Autodesk Fusion 360 part; units mm, degrees
note: some values were not read from the file. Chosen so that the rebuilt part matches the saved one: which bodies a step acts on.
(part 2 of 3)
sketch "Sketch6" plane through (0, 0, 5) normal (0, 0, 1) x (-1, 0, 0)
  arc A0 (-101.6, 90) -> (-98.4, 90) centre (-100, 90) ccw
  line L0 (-101.6, 90) -> (-101.6, 94)
  arc A1 (-98.4, 94) -> (-101.6, 94) centre (-100, 94) ccw
  line L1 (-98.4, 94) -> (-98.4, 90)
  arc A2 (-110, 101.6) -> (-110, 98.4) centre (-110, 100) ccw
  line L2 (-110, 101.6) -> (-106, 101.6)
  arc A3 (-106, 98.4) -> (-106, 101.6) centre (-106, 100) ccw
  line L3 (-106, 98.4) -> (-110, 98.4)
  arc A4 (-90, 98.4) -> (-90, 101.6) centre (-90, 100) ccw
  line L4 (-90, 98.4) -> (-94, 98.4)
  arc A5 (-94, 101.6) -> (-94, 98.4) centre (-94, 100) ccw
  line L5 (-94, 101.6) -> (-90, 101.6)
  circle A6 centre (-100, 100) radius 3
  arc A7 (-98.4, 110) -> (-101.6, 110) centre (-100, 110) ccw
  line L6 (-98.4, 110) -> (-98.4, 106)
  arc A8 (-101.6, 106) -> (-98.4, 106) centre (-100, 106) ccw
  line L7 (-101.6, 106) -> (-101.6, 110)
  arc A9 (-30, -25) -> (-24, -25) centre (-27, -25) ccw
  line L8 (-30, -25) -> (-30, 25)
  arc A10 (-24, 25) -> (-30, 25) centre (-27, 25) ccw
  line L9 (-24, 25) -> (-24, -25)
  arc A11 (-17.7956, -15.5328) -> (-15.5328, -17.7956) centre (-16.6642, -16.6642) ccw
  line L10 (-17.7956, -15.5328) -> (-14.9672, -12.7044)
  arc A12 (-12.7044, -14.9672) -> (-14.9672, -12.7044) centre (-13.8358, -13.8358) ccw
  line L11 (-12.7044, -14.9672) -> (-15.5328, -17.7956)
  line L12 (12.7044, 14.9672) -> (15.5328, 17.7956)
  arc A13 (17.7956, 15.5328) -> (15.5328, 17.7956) centre (16.6642, 16.6642) ccw
  line L13 (17.7956, 15.5328) -> (14.9672, 12.7044)
  arc A14 (12.7044, 14.9672) -> (14.9672, 12.7044) centre (13.8358, 13.8358) ccw
  line L14 (14.9672, -12.7044) -> (17.7956, -15.5328)
  arc A15 (15.5328, -17.7956) -> (17.7956, -15.5328) centre (16.6642, -16.6642) ccw
  line L15 (15.5328, -17.7956) -> (12.7044, -14.9672)
  arc A16 (14.9672, -12.7044) -> (12.7044, -14.9672) centre (13.8358, -13.8358) ccw
  arc A17 (24, -25) -> (30, -25) centre (27, -25) ccw
  line L16 (24, -25) -> (24, 25)
  arc A18 (30, 25) -> (24, 25) centre (27, 25) ccw
  line L17 (30, 25) -> (30, -25)
  line L18 (-14.9672, 12.7044) -> (-17.7956, 15.5328)
  arc A19 (-15.5328, 17.7956) -> (-17.7956, 15.5328) centre (-16.6642, 16.6642) ccw
  line L19 (-15.5328, 17.7956) -> (-12.7044, 14.9672)
  arc A20 (-14.9672, 12.7044) -> (-12.7044, 14.9672) centre (-13.8358, 13.8358) ccw
  line L20 (112.7195, 117.7075) -> (119.1639, 120.4095)
  arc A21 (122.285, 116.8358) -> (119.1639, 120.4095) centre (120.1306, 118.104) ccw
  line L21 (122.285, 116.8358) -> (118.9823, 111.2253)
  arc A22 (116.8279, 109.9935) -> (118.9823, 111.2253) centre (116.8279, 112.4935) ccw
  line L22 (116.8279, 109.9935) -> (113.6861, 109.9935)
  arc A23 (111.1861, 112.4935) -> (113.6861, 109.9935) centre (113.6861, 112.4935) ccw
  line L23 (111.1861, 112.4935) -> (111.1861, 115.4019)
  arc A24 (112.7195, 117.7075) -> (111.1861, 115.4019) centre (113.6861, 115.4019) ccw
  arc A25 (101.6, 110) -> (98.4, 110) centre (100, 110) ccw
  line L24 (101.6, 110) -> (101.6, 106)
  arc A26 (98.4, 106) -> (101.6, 106) centre (100, 106) ccw
  line L25 (98.4, 106) -> (98.4, 110)
  circle A27 centre (100, 100) radius 3
  arc A28 (90, 101.6) -> (90, 98.4) centre (90, 100) ccw
  line L26 (90, 101.6) -> (94, 101.6)
  arc A29 (94, 98.4) -> (94, 101.6) centre (94, 100) ccw
  line L27 (94, 98.4) -> (90, 98.4)
  arc A30 (110, 98.4) -> (110, 101.6) centre (110, 100) ccw
  line L28 (110, 98.4) -> (106, 98.4)
  arc A31 (106, 101.6) -> (106, 98.4) centre (106, 100) ccw
  line L29 (106, 101.6) -> (110, 101.6)
  arc A32 (98.4, 90) -> (101.6, 90) centre (100, 90) ccw
  line L30 (98.4, 90) -> (98.4, 94)
  arc A33 (101.6, 94) -> (98.4, 94) centre (100, 94) ccw
  line L31 (101.6, 94) -> (101.6, 90)
  arc A34 (101.6, -90) -> (98.4, -90) centre (100, -90) ccw
  line L32 (101.6, -90) -> (101.6, -94)
  arc A35 (98.4, -94) -> (101.6, -94) centre (100, -94) ccw
  line L33 (98.4, -94) -> (98.4, -90)
  arc A36 (110, -101.6) -> (110, -98.4) centre (110, -100) ccw
  line L34 (110, -101.6) -> (106, -101.6)
  arc A37 (106, -98.4) -> (106, -101.6) centre (106, -100) ccw
  line L35 (106, -98.4) -> (110, -98.4)
  arc A38 (90, -98.4) -> (90, -101.6) centre (90, -100) ccw
  line L36 (90, -98.4) -> (94, -98.4)
  arc A39 (94, -101.6) -> (94, -98.4) centre (94, -100) ccw
  line L37 (94, -101.6) -> (90, -101.6)
  circle A40 centre (100, -100) radius 3
  arc A41 (98.4, -110) -> (101.6, -110) centre (100, -110) ccw
  line L38 (98.4, -110) -> (98.4, -106)
  arc A42 (101.6, -106) -> (98.4, -106) centre (100, -106) ccw
  line L39 (101.6, -106) -> (101.6, -110)
  line L40 (118.9823, -111.2253) -> (122.285, -116.8358)
  arc A43 (119.1639, -120.4095) -> (122.285, -116.8358) centre (120.1306, -118.104) ccw
  line L41 (119.1639, -120.4095) -> (112.7195, -117.7075)
  arc A44 (111.1861, -115.4019) -> (112.7195, -117.7075) centre (113.6861, -115.4019) ccw
  line L42 (111.1861, -115.4019) -> (111.1861, -112.4935)
  arc A45 (113.6861, -109.9935) -> (111.1861, -112.4935) centre (113.6861, -112.4935) ccw
  line L43 (113.6861, -109.9935) -> (116.8279, -109.9935)
  arc A46 (118.9823, -111.2253) -> (116.8279, -109.9935) centre (116.8279, -112.4935) ccw
  arc A47 (-101.6, -110) -> (-98.4, -110) centre (-100, -110) ccw
  line L44 (-101.6, -110) -> (-101.6, -106)
  arc A48 (-98.4, -106) -> (-101.6, -106) centre (-100, -106) ccw
  line L45 (-98.4, -106) -> (-98.4, -110)
  circle A49 centre (-100, -100) radius 3
  arc A50 (-90, -101.6) -> (-90, -98.4) centre (-90, -100) ccw
  line L46 (-90, -101.6) -> (-94, -101.6)
  arc A51 (-94, -98.4) -> (-94, -101.6) centre (-94, -100) ccw
  line L47 (-94, -98.4) -> (-90, -98.4)
  arc A52 (-110, -98.4) -> (-110, -101.6) centre (-110, -100) ccw
  line L48 (-110, -98.4) -> (-106, -98.4)
  arc A53 (-106, -101.6) -> (-106, -98.4) centre (-106, -100) ccw
  line L49 (-106, -101.6) -> (-110, -101.6)
  arc A54 (-98.4, -90) -> (-101.6, -90) centre (-100, -90) ccw
  line L50 (-98.4, -90) -> (-98.4, -94)
  arc A55 (-101.6, -94) -> (-98.4, -94) centre (-100, -94) ccw
  line L51 (-101.6, -94) -> (-101.6, -90)
  line L52 (-116.8279, -109.9935) -> (-113.6861, -109.9935)
  arc A56 (-111.1861, -112.4935) -> (-113.6861, -109.9935) centre (-113.6861, -112.4935) ccw
  line L53 (-111.1861, -112.4935) -> (-111.1861, -115.4019)
  arc A57 (-112.7195, -117.7075) -> (-111.1861, -115.4019) centre (-113.6861, -115.4019) ccw
  line L54 (-112.7195, -117.7075) -> (-119.1639, -120.4095)
  arc A58 (-122.285, -116.8358) -> (-119.1639, -120.4095) centre (-120.1306, -118.104) ccw
  line L55 (-122.285, -116.8358) -> (-118.9823, -111.2253)
  arc A59 (-116.8279, -109.9935) -> (-118.9823, -111.2253) centre (-116.8279, -112.4935) ccw
  line L56 (-118.9823, 111.2253) -> (-122.285, 116.8358)
  arc A60 (-119.1639, 120.4095) -> (-122.285, 116.8358) centre (-120.1306, 118.104) ccw
  line L57 (-119.1639, 120.4095) -> (-112.7195, 117.7075)
  arc A61 (-111.1861, 115.4019) -> (-112.7195, 117.7075) centre (-113.6861, 115.4019) ccw
  line L58 (-111.1861, 115.4019) -> (-111.1861, 112.4935)
  arc A62 (-113.6861, 109.9935) -> (-111.1861, 112.4935) centre (-113.6861, 112.4935) ccw
  line L59 (-113.6861, 109.9935) -> (-116.8279, 109.9935)
  arc A63 (-118.9823, 111.2253) -> (-116.8279, 109.9935) centre (-116.8279, 112.4935) ccw
  arc A64 (16.6527, -80.0321) -> (19.3611, -77.7595) centre (16.8706, -77.5416) ccw
  line L60 (19.3611, -77.7595) -> (21.3355, -55.1918)
  arc A65 (29.6477, -51.8989) -> (21.3355, -55.1918) centre (26.3165, -55.6276) ccw
  line L61 (29.6477, -51.8989) -> (81.7303, -98.4286)
  arc A66 (86.4985, -105.2878) -> (81.7303, -98.4286) centre (69.7381, -111.852) ccw
  arc A67 (86.4985, -105.2878) -> (94.5518, -113.4375) centre (100, -100) ccw
  line L62 (94.5518, -113.4375) -> (119.1307, -123.403)
  arc A68 (119.1307, -123.403) -> (125.4028, -116.3824) centre (121.0094, -118.7694) ccw
  line L63 (125.4028, -116.3824) -> (112.7409, -93.0776)
  arc A69 (112.7409, -93.0776) -> (103.7386, -85.9903) centre (100, -100) ccw
  arc A70 (96.3875, -82.0222) -> (103.7386, -85.9903) centre (108.3797, -68.5989) ccw
  line L64 (96.3875, -82.0222) -> (44.6753, -35.8235)
  arc A71 (38, -20.9087) -> (44.6753, -35.8235) centre (58, -20.9087) ccw
  line L65 (38, -20.9087) -> (38, 20.9087)
  arc A72 (44.6753, 35.8235) -> (38, 20.9087) centre (58, 20.9087) ccw
  line L66 (44.6753, 35.8235) -> (96.3875, 82.0222)
  arc A73 (103.7386, 85.9903) -> (96.3875, 82.0222) centre (108.3797, 68.5989) ccw
  arc A74 (103.7386, 85.9903) -> (112.7409, 93.0776) centre (100, 100) ccw
  line L67 (112.7409, 93.0776) -> (125.4028, 116.3824)
  arc A75 (125.4028, 116.3824) -> (119.1307, 123.403) centre (121.0094, 118.7694) ccw
  line L68 (119.1307, 123.403) -> (94.5518, 113.4375)
  arc A76 (94.5518, 113.4375) -> (86.4985, 105.2878) centre (100, 100) ccw
  arc A77 (81.7303, 98.4286) -> (86.4985, 105.2878) centre (69.7381, 111.852) ccw
  line L69 (81.7303, 98.4286) -> (29.156, 51.4596)
  arc A78 (20.8759, 54.4751) -> (29.156, 51.4596) centre (25.8248, 55.1883) ccw
  line L70 (20.8759, 54.4751) -> (16.1217, 87.466)
  arc A79 (16.1217, 87.466) -> (14.4465, 90.5321) centre (11.1729, 86.7528) ccw
  line L71 (14.4465, 90.5321) -> (10.4093, 94.0293)
  arc A80 (10.4093, 94.0293) -> (7.1356, 95.25) centre (7.1356, 90.25) ccw
  line L72 (7.1356, 95.25) -> (-7.1356, 95.25)
  arc A81 (-7.1356, 95.25) -> (-10.4093, 94.0293) centre (-7.1356, 90.25) ccw
  line L73 (-10.4093, 94.0293) -> (-14.4465, 90.5321)
  arc A82 (-14.4465, 90.5321) -> (-16.1217, 87.466) centre (-11.1729, 86.7528) ccw
  line L74 (-16.1217, 87.466) -> (-20.8759, 54.4751)
  arc A83 (-29.156, 51.4596) -> (-20.8759, 54.4751) centre (-25.8248, 55.1883) ccw
  line L75 (-29.156, 51.4596) -> (-81.7303, 98.4286)
  arc A84 (-86.4985, 105.2878) -> (-81.7303, 98.4286) centre (-69.7381, 111.852) ccw
  arc A85 (-86.4985, 105.2878) -> (-94.5518, 113.4375) centre (-100, 100) ccw
  line L76 (-94.5518, 113.4375) -> (-119.1307, 123.403)
  arc A86 (-119.1307, 123.403) -> (-125.4028, 116.3824) centre (-121.0094, 118.7694) ccw
  line L77 (-125.4028, 116.3824) -> (-112.7409, 93.0776)
  arc A87 (-112.7409, 93.0776) -> (-103.7386, 85.9903) centre (-100, 100) ccw
  arc A88 (-96.3875, 82.0222) -> (-103.7386, 85.9903) centre (-108.3797, 68.5989) ccw
  line L78 (-96.3875, 82.0222) -> (-44.6753, 35.8235)
  arc A89 (-38, 20.9087) -> (-44.6753, 35.8235) centre (-58, 20.9087) ccw
  line L79 (-38, 20.9087) -> (-38, -20.9087)
  arc A90 (-44.6753, -35.8235) -> (-38, -20.9087) centre (-58, -20.9087) ccw
  line L80 (-44.6753, -35.8235) -> (-96.3875, -82.0222)
  arc A91 (-103.7386, -85.9903) -> (-96.3875, -82.0222) centre (-108.3797, -68.5989) ccw
  arc A92 (-103.7386, -85.9903) -> (-112.7409, -93.0776) centre (-100, -100) ccw
  line L81 (-112.7409, -93.0776) -> (-125.4028, -116.3824)
  arc A93 (-125.4028, -116.3824) -> (-119.1307, -123.403) centre (-121.0094, -118.7694) ccw
  line L82 (-119.1307, -123.403) -> (-94.5518, -113.4375)
  arc A94 (-94.5518, -113.4375) -> (-86.4985, -105.2878) centre (-100, -100) ccw
  arc A95 (-81.7303, -98.4286) -> (-86.4985, -105.2878) centre (-69.7381, -111.852) ccw
  line L83 (-81.7303, -98.4286) -> (-29.6477, -51.8989)
  arc A96 (-21.3355, -55.1918) -> (-29.6477, -51.8989) centre (-26.3165, -55.6276) ccw
  line L84 (-21.3355, -55.1918) -> (-19.3611, -77.7595)
  arc A97 (-19.3611, -77.7595) -> (-16.6527, -80.0321) centre (-16.8706, -77.5416) ccw
  line L85 (-16.6527, -80.0321) -> (-12.2821, -79.6497)
  arc A98 (-12.2821, -79.6497) -> (-10.0175, -77.4546) centre (-12.5, -77.1592) ccw
  arc A99 (-7.535, -75.25) -> (-10.0175, -77.4546) centre (-7.535, -77.75) ccw
  line L86 (-7.535, -75.25) -> (7.535, -75.25)
  arc A100 (10.0175, -77.4546) -> (7.535, -75.25) centre (7.535, -77.75) ccw
  arc A101 (10.0175, -77.4546) -> (12.2821, -79.6497) centre (12.5, -77.1592) ccw
  line L87 (12.2821, -79.6497) -> (16.6527, -80.0321)
  line L88 (26, 35.4) -> (18, 35.4)
  arc A102 (18, 38.6) -> (18, 35.4) centre (18, 37) ccw
  line L89 (18, 38.6) -> (26, 38.6)
  arc A103 (26, 35.4) -> (26, 38.6) centre (26, 37) ccw
  circle A104 centre (14.8248, -75.7565) radius 1.6
  line L90 (-5, -61.3002) -> (5, -61.3002)
  arc A105 (5, -71.3002) -> (5, -61.3002) centre (5, -66.3002) ccw
  line L91 (5, -71.3002) -> (-5, -71.3002)
  arc A106 (-5, -61.3002) -> (-5, -71.3002) centre (-5, -66.3002) ccw
  circle A107 centre (16.4789, -56.85) radius 1.6
  line L92 (10, 39) -> (10, 36)
  arc A108 (4, 30) -> (10, 36) centre (4, 36) ccw
  line L93 (4, 30) -> (-4, 30)
  arc A109 (-10, 36) -> (-4, 30) centre (-4, 36) ccw
  line L94 (-10, 36) -> (-10, 39)
  arc A110 (-4, 45) -> (-10, 39) centre (-4, 39) ccw
  line L95 (-4, 45) -> (4, 45)
  arc A111 (10, 39) -> (4, 45) centre (4, 39) ccw
  line L96 (-26, 38.6) -> (-18, 38.6)
  arc A112 (-18, 35.4) -> (-18, 38.6) centre (-18, 37) ccw
  line L97 (-18, 35.4) -> (-26, 35.4)
  arc A113 (-26, 38.6) -> (-26, 35.4) centre (-26, 37) ccw
  circle A114 centre (-14.8248, -75.7565) radius 1.6
  line L98 (-12.5, -35.4) -> (12.5, -35.4)
  arc A115 (12.5, -38.6) -> (12.5, -35.4) centre (12.5, -37) ccw
  line L99 (12.5, -38.6) -> (-12.5, -38.6)
  arc A116 (-12.5, -35.4) -> (-12.5, -38.6) centre (-12.5, -37) ccw
  circle A117 centre (-16.4789, -56.85) radius 1.6
  line L100 (6, 80.25) -> (6, 60.25)
  arc A118 (-6, 60.25) -> (6, 60.25) centre (0, 60.25) ccw
  line L101 (-6, 60.25) -> (-6, 80.25)
  arc A119 (6, 80.25) -> (-6, 80.25) centre (0, 80.25) ccw
  line L102 (0, -61.3002) -> (0, -38.6) construction
  line L103 (5, -52.8369) -> (-5, -52.8369)
  line L104 (-5, -52.8369) -> (0, -44.1766)
  line L105 (5, -52.8369) -> (0, -44.1766)
  line L106 (2.5, -48.5067) -> (0, -49.9501)
  line L107 (-2.5, -48.5067) -> (0, -49.9501)
  line L108 (0, -52.8369) -> (0, -49.9501)
  dimension "d99" = 10
  constraint midpoint L90 L102.start
  constraint midpoint L99 L102.end
  constraint perpendicular L102 L103
  constraint coincident L102 L104.end
  constraint equal L103 L104
  constraint equal L103 L105
  constraint midpoint L105 L106.start
  constraint coincident L102 L106.end
  constraint perpendicular L105 L106
  constraint midpoint L104 L107.start
  constraint midpoint L103 L108.start
  constraint midpoint L102 L106.end
  measures "d99" distance of L103.start L103.end
extrude "Extrude6" cut sketch "Sketch6" against normal blind 5 contours L103 L105 L106 L108 | L103 L104 L107 L108 | L104 L105 L106 L107 bodies 2
chamfer "Chamfer2" distance 2 angle 45 3 edges at (-5, 52.8369, 2.5) (5, 52.8369, 2.5) (0, 44.1766, 2.5) on bodies 2
sketch "Sketch7" plane through (0, 0, 5) normal (0, 0, 1) x (-1, 0, 0)
  line L0 (6, 80.25) -> (6, 60.25)
  arc A0 (-6, 60.25) -> (6, 60.25) centre (0, 60.25) ccw
  line L1 (-6, 60.25) -> (-6, 80.25)
  arc A1 (6, 80.25) -> (-6, 80.25) centre (0, 80.25) ccw
  circle A2 centre (-16.4789, -56.85) radius 1.6
  line L2 (-12.5, -35.4) -> (12.5, -35.4)
  arc A3 (12.5, -38.6) -> (12.5, -35.4) centre (12.5, -37) ccw
  line L3 (12.5, -38.6) -> (-12.5, -38.6)
  arc A4 (-12.5, -35.4) -> (-12.5, -38.6) centre (-12.5, -37) ccw
  circle A5 centre (-14.8248, -75.7565) radius 1.6
  line L4 (-26, 38.6) -> (-18, 38.6)
  arc A6 (-18, 35.4) -> (-18, 38.6) centre (-18, 37) ccw
  line L5 (-18, 35.4) -> (-26, 35.4)
  arc A7 (-26, 38.6) -> (-26, 35.4) centre (-26, 37) ccw
  line L6 (10, 39) -> (10, 36)
  arc A8 (4, 30) -> (10, 36) centre (4, 36) ccw
  line L7 (4, 30) -> (-4, 30)
  arc A9 (-10, 36) -> (-4, 30) centre (-4, 36) ccw
  line L8 (-10, 36) -> (-10, 39)
  arc A10 (-4, 45) -> (-10, 39) centre (-4, 39) ccw
  line L9 (-4, 45) -> (4, 45)
  arc A11 (10, 39) -> (4, 45) centre (4, 39) ccw
  circle A12 centre (16.4789, -56.85) radius 1.6
  line L10 (-5, -61.3002) -> (5, -61.3002)
  arc A13 (5, -71.3002) -> (5, -61.3002) centre (5, -66.3002) ccw
  line L11 (5, -71.3002) -> (-5, -71.3002)
  arc A14 (-5, -61.3002) -> (-5, -71.3002) centre (-5, -66.3002) ccw
  circle A15 centre (14.8248, -75.7565) radius 1.6
  line L12 (26, 35.4) -> (18, 35.4)
  arc A16 (18, 38.6) -> (18, 35.4) centre (18, 37) ccw
  line L13 (18, 38.6) -> (26, 38.6)
  arc A17 (26, 35.4) -> (26, 38.6) centre (26, 37) ccw
  arc A18 (16.6527, -80.0321) -> (19.3611, -77.7595) centre (16.8706, -77.5416) ccw
  line L14 (19.3611, -77.7595) -> (21.3355, -55.1918)
  arc A19 (29.6477, -51.8989) -> (21.3355, -55.1918) centre (26.3165, -55.6276) ccw
  line L15 (29.6477, -51.8989) -> (81.7303, -98.4286)
  arc A20 (86.4985, -105.2878) -> (81.7303, -98.4286) centre (69.7381, -111.852) ccw
  arc A21 (86.4985, -105.2878) -> (94.5518, -113.4375) centre (100, -100) ccw
  line L16 (94.5518, -113.4375) -> (119.1307, -123.403)
  arc A22 (119.1307, -123.403) -> (125.4028, -116.3824) centre (121.0094, -118.7694) ccw
  line L17 (125.4028, -116.3824) -> (112.7409, -93.0776)
  arc A23 (112.7409, -93.0776) -> (103.7386, -85.9903) centre (100, -100) ccw
  arc A24 (96.3875, -82.0222) -> (103.7386, -85.9903) centre (108.3797, -68.5989) ccw
  line L18 (96.3875, -82.0222) -> (44.6753, -35.8235)
  arc A25 (38, -20.9087) -> (44.6753, -35.8235) centre (58, -20.9087) ccw
  line L19 (38, -20.9087) -> (38, 20.9087)
  arc A26 (44.6753, 35.8235) -> (38, 20.9087) centre (58, 20.9087) ccw
  line L20 (44.6753, 35.8235) -> (96.3875, 82.0222)
  arc A27 (103.7386, 85.9903) -> (96.3875, 82.0222) centre (108.3797, 68.5989) ccw
  arc A28 (103.7386, 85.9903) -> (112.7409, 93.0776) centre (100, 100) ccw
  line L21 (112.7409, 93.0776) -> (125.4028, 116.3824)
  arc A29 (125.4028, 116.3824) -> (119.1307, 123.403) centre (121.0094, 118.7694) ccw
  line L22 (119.1307, 123.403) -> (94.5518, 113.4375)
  arc A30 (94.5518, 113.4375) -> (86.4985, 105.2878) centre (100, 100) ccw
  arc A31 (81.7303, 98.4286) -> (86.4985, 105.2878) centre (69.7381, 111.852) ccw
  line L23 (81.7303, 98.4286) -> (29.156, 51.4596)
  arc A32 (20.8759, 54.4751) -> (29.156, 51.4596) centre (25.8248, 55.1883) ccw
  line L24 (20.8759, 54.4751) -> (16.1217, 87.466)
  arc A33 (16.1217, 87.466) -> (14.4465, 90.5321) centre (11.1729, 86.7528) ccw
  line L25 (14.4465, 90.5321) -> (10.4093, 94.0293)
  arc A34 (10.4093, 94.0293) -> (7.1356, 95.25) centre (7.1356, 90.25) ccw
  line L26 (7.1356, 95.25) -> (-7.1356, 95.25)
  arc A35 (-7.1356, 95.25) -> (-10.4093, 94.0293) centre (-7.1356, 90.25) ccw
  line L27 (-10.4093, 94.0293) -> (-14.4465, 90.5321)
  arc A36 (-14.4465, 90.5321) -> (-16.1217, 87.466) centre (-11.1729, 86.7528) ccw
  line L28 (-16.1217, 87.466) -> (-20.8759, 54.4751)
  arc A37 (-29.156, 51.4596) -> (-20.8759, 54.4751) centre (-25.8248, 55.1883) ccw
  line L29 (-29.156, 51.4596) -> (-81.7303, 98.4286)
  arc A38 (-86.4985, 105.2878) -> (-81.7303, 98.4286) centre (-69.7381, 111.852) ccw
  arc A39 (-86.4985, 105.2878) -> (-94.5518, 113.4375) centre (-100, 100) ccw
  line L30 (-94.5518, 113.4375) -> (-119.1307, 123.403)
  arc A40 (-119.1307, 123.403) -> (-125.4028, 116.3824) centre (-121.0094, 118.7694) ccw
  line L31 (-125.4028, 116.3824) -> (-112.7409, 93.0776)
  arc A41 (-112.7409, 93.0776) -> (-103.7386, 85.9903) centre (-100, 100) ccw
  arc A42 (-96.3875, 82.0222) -> (-103.7386, 85.9903) centre (-108.3797, 68.5989) ccw
  line L32 (-96.3875, 82.0222) -> (-44.6753, 35.8235)
  arc A43 (-38, 20.9087) -> (-44.6753, 35.8235) centre (-58, 20.9087) ccw
  line L33 (-38, 20.9087) -> (-38, -20.9087)
  arc A44 (-44.6753, -35.8235) -> (-38, -20.9087) centre (-58, -20.9087) ccw
  line L34 (-44.6753, -35.8235) -> (-96.3875, -82.0222)
  arc A45 (-103.7386, -85.9903) -> (-96.3875, -82.0222) centre (-108.3797, -68.5989) ccw
  arc A46 (-103.7386, -85.9903) -> (-112.7409, -93.0776) centre (-100, -100) ccw
  line L35 (-112.7409, -93.0776) -> (-125.4028, -116.3824)
  arc A47 (-125.4028, -116.3824) -> (-119.1307, -123.403) centre (-121.0094, -118.7694) ccw
  line L36 (-119.1307, -123.403) -> (-94.5518, -113.4375)
  arc A48 (-94.5518, -113.4375) -> (-86.4985, -105.2878) centre (-100, -100) ccw
  arc A49 (-81.7303, -98.4286) -> (-86.4985, -105.2878) centre (-69.7381, -111.852) ccw
  line L37 (-81.7303, -98.4286) -> (-29.6477, -51.8989)
  arc A50 (-21.3355, -55.1918) -> (-29.6477, -51.8989) centre (-26.3165, -55.6276) ccw
  line L38 (-21.3355, -55.1918) -> (-19.3611, -77.7595)
  arc A51 (-19.3611, -77.7595) -> (-16.6527, -80.0321) centre (-16.8706, -77.5416) ccw
  line L39 (-16.6527, -80.0321) -> (-12.2821, -79.6497)
  arc A52 (-12.2821, -79.6497) -> (-10.0175, -77.4546) centre (-12.5, -77.1592) ccw
  arc A53 (-7.535, -75.25) -> (-10.0175, -77.4546) centre (-7.535, -77.75) ccw
  line L40 (-7.535, -75.25) -> (7.535, -75.25)
  arc A54 (10.0175, -77.4546) -> (7.535, -75.25) centre (7.535, -77.75) ccw
  arc A55 (10.0175, -77.4546) -> (12.2821, -79.6497) centre (12.5, -77.1592) ccw
  line L41 (12.2821, -79.6497) -> (16.6527, -80.0321)
  line L42 (-118.9823, 111.2253) -> (-122.285, 116.8358)
  arc A56 (-119.1639, 120.4095) -> (-122.285, 116.8358) centre (-120.1306, 118.104) ccw
  line L43 (-119.1639, 120.4095) -> (-112.7195, 117.7075)
  arc A57 (-111.1861, 115.4019) -> (-112.7195, 117.7075) centre (-113.6861, 115.4019) ccw
  line L44 (-111.1861, 115.4019) -> (-111.1861, 112.4935)
  arc A58 (-113.6861, 109.9935) -> (-111.1861, 112.4935) centre (-113.6861, 112.4935) ccw
  line L45 (-113.6861, 109.9935) -> (-116.8279, 109.9935)
  arc A59 (-118.9823, 111.2253) -> (-116.8279, 109.9935) centre (-116.8279, 112.4935) ccw
  line L46 (-116.8279, -109.9935) -> (-113.6861, -109.9935)
  arc A60 (-111.1861, -112.4935) -> (-113.6861, -109.9935) centre (-113.6861, -112.4935) ccw
  line L47 (-111.1861, -112.4935) -> (-111.1861, -115.4019)
  arc A61 (-112.7195, -117.7075) -> (-111.1861, -115.4019) centre (-113.6861, -115.4019) ccw
  line L48 (-112.7195, -117.7075) -> (-119.1639, -120.4095)
  arc A62 (-122.285, -116.8358) -> (-119.1639, -120.4095) centre (-120.1306, -118.104) ccw
  line L49 (-122.285, -116.8358) -> (-118.9823, -111.2253)
  arc A63 (-116.8279, -109.9935) -> (-118.9823, -111.2253) centre (-116.8279, -112.4935) ccw
  arc A64 (-98.4, -90) -> (-101.6, -90) centre (-100, -90) ccw
  line L50 (-98.4, -90) -> (-98.4, -94)
  arc A65 (-101.6, -94) -> (-98.4, -94) centre (-100, -94) ccw
  line L51 (-101.6, -94) -> (-101.6, -90)
  arc A66 (-110, -98.4) -> (-110, -101.6) centre (-110, -100) ccw
  line L52 (-110, -98.4) -> (-106, -98.4)
  arc A67 (-106, -101.6) -> (-106, -98.4) centre (-106, -100) ccw
  line L53 (-106, -101.6) -> (-110, -101.6)
  arc A68 (-90, -101.6) -> (-90, -98.4) centre (-90, -100) ccw
  line L54 (-90, -101.6) -> (-94, -101.6)
  arc A69 (-94, -98.4) -> (-94, -101.6) centre (-94, -100) ccw
  line L55 (-94, -98.4) -> (-90, -98.4)
  circle A70 centre (-100, -100) radius 3
  arc A71 (-101.6, -110) -> (-98.4, -110) centre (-100, -110) ccw
  line L56 (-101.6, -110) -> (-101.6, -106)
  arc A72 (-98.4, -106) -> (-101.6, -106) centre (-100, -106) ccw
  line L57 (-98.4, -106) -> (-98.4, -110)
  line L58 (118.9823, -111.2253) -> (122.285, -116.8358)
  arc A73 (119.1639, -120.4095) -> (122.285, -116.8358) centre (120.1306, -118.104) ccw
  line L59 (119.1639, -120.4095) -> (112.7195, -117.7075)
  arc A74 (111.1861, -115.4019) -> (112.7195, -117.7075) centre (113.6861, -115.4019) ccw
  line L60 (111.1861, -115.4019) -> (111.1861, -112.4935)
  arc A75 (113.6861, -109.9935) -> (111.1861, -112.4935) centre (113.6861, -112.4935) ccw
  line L61 (113.6861, -109.9935) -> (116.8279, -109.9935)
  arc A76 (118.9823, -111.2253) -> (116.8279, -109.9935) centre (116.8279, -112.4935) ccw
  arc A77 (98.4, -110) -> (101.6, -110) centre (100, -110) ccw
  line L62 (98.4, -110) -> (98.4, -106)
  arc A78 (101.6, -106) -> (98.4, -106) centre (100, -106) ccw
  line L63 (101.6, -106) -> (101.6, -110)
  circle A79 centre (100, -100) radius 3
  arc A80 (90, -98.4) -> (90, -101.6) centre (90, -100) ccw
  line L64 (90, -98.4) -> (94, -98.4)
  arc A81 (94, -101.6) -> (94, -98.4) centre (94, -100) ccw
  line L65 (94, -101.6) -> (90, -101.6)
  arc A82 (110, -101.6) -> (110, -98.4) centre (110, -100) ccw
  line L66 (110, -101.6) -> (106, -101.6)
  arc A83 (106, -98.4) -> (106, -101.6) centre (106, -100) ccw
  line L67 (106, -98.4) -> (110, -98.4)
  arc A84 (101.6, -90) -> (98.4, -90) centre (100, -90) ccw
  line L68 (101.6, -90) -> (101.6, -94)
  arc A85 (98.4, -94) -> (101.6, -94) centre (100, -94) ccw
  line L69 (98.4, -94) -> (98.4, -90)
  arc A86 (98.4, 90) -> (101.6, 90) centre (100, 90) ccw
  line L70 (98.4, 90) -> (98.4, 94)
  arc A87 (101.6, 94) -> (98.4, 94) centre (100, 94) ccw
  line L71 (101.6, 94) -> (101.6, 90)
  arc A88 (110, 98.4) -> (110, 101.6) centre (110, 100) ccw
  line L72 (110, 98.4) -> (106, 98.4)
  arc A89 (106, 101.6) -> (106, 98.4) centre (106, 100) ccw
  line L73 (106, 101.6) -> (110, 101.6)
  arc A90 (90, 101.6) -> (90, 98.4) centre (90, 100) ccw
  line L74 (90, 101.6) -> (94, 101.6)
  arc A91 (94, 98.4) -> (94, 101.6) centre (94, 100) ccw
  line L75 (94, 98.4) -> (90, 98.4)
  circle A92 centre (100, 100) radius 3
  arc A93 (101.6, 110) -> (98.4, 110) centre (100, 110) ccw
  line L76 (101.6, 110) -> (101.6, 106)
  arc A94 (98.4, 106) -> (101.6, 106) centre (100, 106) ccw
  line L77 (98.4, 106) -> (98.4, 110)
  line L78 (112.7195, 117.7075) -> (119.1639, 120.4095)
  arc A95 (122.285, 116.8358) -> (119.1639, 120.4095) centre (120.1306, 118.104) ccw
  line L79 (122.285, 116.8358) -> (118.9823, 111.2253)
  arc A96 (116.8279, 109.9935) -> (118.9823, 111.2253) centre (116.8279, 112.4935) ccw
  line L80 (116.8279, 109.9935) -> (113.6861, 109.9935)
  arc A97 (111.1861, 112.4935) -> (113.6861, 109.9935) centre (113.6861, 112.4935) ccw
  line L81 (111.1861, 112.4935) -> (111.1861, 115.4019)
  arc A98 (112.7195, 117.7075) -> (111.1861, 115.4019) centre (113.6861, 115.4019) ccw
  line L82 (-14.9672, 12.7044) -> (-17.7956, 15.5328)
  arc A99 (-15.5328, 17.7956) -> (-17.7956, 15.5328) centre (-16.6642, 16.6642) ccw
  line L83 (-15.5328, 17.7956) -> (-12.7044, 14.9672)
  arc A100 (-14.9672, 12.7044) -> (-12.7044, 14.9672) centre (-13.8358, 13.8358) ccw
  arc A101 (24, -25) -> (30, -25) centre (27, -25) ccw
  line L84 (24, -25) -> (24, 25)
  arc A102 (30, 25) -> (24, 25) centre (27, 25) ccw
  line L85 (30, 25) -> (30, -25)
  line L86 (14.9672, -12.7044) -> (17.7956, -15.5328)
  arc A103 (15.5328, -17.7956) -> (17.7956, -15.5328) centre (16.6642, -16.6642) ccw
  line L87 (15.5328, -17.7956) -> (12.7044, -14.9672)
  arc A104 (14.9672, -12.7044) -> (12.7044, -14.9672) centre (13.8358, -13.8358) ccw
  line L88 (12.7044, 14.9672) -> (15.5328, 17.7956)
  arc A105 (17.7956, 15.5328) -> (15.5328, 17.7956) centre (16.6642, 16.6642) ccw
  line L89 (17.7956, 15.5328) -> (14.9672, 12.7044)
  arc A106 (12.7044, 14.9672) -> (14.9672, 12.7044) centre (13.8358, 13.8358) ccw
  arc A107 (-17.7956, -15.5328) -> (-15.5328, -17.7956) centre (-16.6642, -16.6642) ccw
  line L90 (-17.7956, -15.5328) -> (-14.9672, -12.7044)
  arc A108 (-12.7044, -14.9672) -> (-14.9672, -12.7044) centre (-13.8358, -13.8358) ccw
  line L91 (-12.7044, -14.9672) -> (-15.5328, -17.7956)
  arc A109 (-30, -25) -> (-24, -25) centre (-27, -25) ccw
  line L92 (-30, -25) -> (-30, 25)
  arc A110 (-24, 25) -> (-30, 25) centre (-27, 25) ccw
  line L93 (-24, 25) -> (-24, -25)
  arc A111 (-98.4, 110) -> (-101.6, 110) centre (-100, 110) ccw
  line L94 (-98.4, 110) -> (-98.4, 106)
  arc A112 (-101.6, 106) -> (-98.4, 106) centre (-100, 106) ccw
  line L95 (-101.6, 106) -> (-101.6, 110)
  circle A113 centre (-100, 100) radius 3
  arc A114 (-90, 98.4) -> (-90, 101.6) centre (-90, 100) ccw
  line L96 (-90, 98.4) -> (-94, 98.4)
  arc A115 (-94, 101.6) -> (-94, 98.4) centre (-94, 100) ccw
  line L97 (-94, 101.6) -> (-90, 101.6)
  arc A116 (-110, 101.6) -> (-110, 98.4) centre (-110, 100) ccw
  line L98 (-110, 101.6) -> (-106, 101.6)
  arc A117 (-106, 98.4) -> (-106, 101.6) centre (-106, 100) ccw
  line L99 (-106, 98.4) -> (-110, 98.4)
  arc A118 (-101.6, 90) -> (-98.4, 90) centre (-100, 90) ccw
  line L100 (-101.6, 90) -> (-101.6, 94)
  arc A119 (-98.4, 94) -> (-101.6, 94) centre (-100, 94) ccw
  line L101 (-98.4, 94) -> (-98.4, 90)
  line L102 (1, -45.9087) -> (4, -51.1048)
  line L103 (4, -51.1048) -> (3, -52.8369)
  line L104 (3, -52.8369) -> (-3, -52.8369)
  line L105 (-3, -52.8369) -> (-4, -51.1048)
  line L106 (-4, -51.1048) -> (-1, -45.9087)
  line L107 (-1, -45.9087) -> (1, -45.9087)
  line L108 (-8.6603, -5) -> (0, -10)
  line L109 (0, -10) -> (8.6603, -5)
  line L110 (8.6603, -5) -> (8.6603, 5)
  line L111 (8.6603, 5) -> (0, 10)
  line L112 (0, 10) -> (-8.6603, 5)
  line L113 (-8.6603, 5) -> (-8.6603, -5)
  line L114 (0, -10) -> (0, 0) construction
  line L115 (1.6, -11) -> (1.6, -9)
  arc A120 (1.6, -9) -> (-1.6, -9) centre (0, -9) ccw
  line L116 (-1.6, -9) -> (-1.6, -11)
  arc A121 (-1.6, -11) -> (1.6, -11) centre (0, -11) ccw
  line L117 (0, -11) -> (0, -9) construction
  arc A122 (8.7263, -6.8856) -> (10.3263, -4.1144) centre (9.5263, -5.5) ccw
  line L118 (10.3263, -4.1144) -> (8.5942, -3.1144)
  line L119 (6.9942, -5.8856) -> (8.7263, -6.8856)
  arc A123 (8.5942, -3.1144) -> (6.9942, -5.8856) centre (7.7942, -4.5) ccw
  arc A124 (10.3263, 4.1144) -> (8.7263, 6.8856) centre (9.5263, 5.5) ccw
  line L120 (8.7263, 6.8856) -> (6.9942, 5.8856)
  line L121 (8.5942, 3.1144) -> (10.3263, 4.1144)
  arc A125 (6.9942, 5.8856) -> (8.5942, 3.1144) centre (7.7942, 4.5) ccw
  arc A126 (1.6, 11) -> (-1.6, 11) centre (0, 11) ccw
  line L122 (-1.6, 11) -> (-1.6, 9)
  line L123 (1.6, 9) -> (1.6, 11)
  arc A127 (-1.6, 9) -> (1.6, 9) centre (0, 9) ccw
  arc A128 (-8.7263, 6.8856) -> (-10.3263, 4.1144) centre (-9.5263, 5.5) ccw
  line L124 (-10.3263, 4.1144) -> (-8.5942, 3.1144)
  line L125 (-6.9942, 5.8856) -> (-8.7263, 6.8856)
  arc A129 (-8.5942, 3.1144) -> (-6.9942, 5.8856) centre (-7.7942, 4.5) ccw
  arc A130 (-10.3263, -4.1144) -> (-8.7263, -6.8856) centre (-9.5263, -5.5) ccw
  line L126 (-8.7263, -6.8856) -> (-6.9942, -5.8856)
  line L127 (-8.5942, -3.1144) -> (-10.3263, -4.1144)
  arc A131 (-6.9942, -5.8856) -> (-8.5942, -3.1144) centre (-7.7942, -4.5) ccw
  point P0 (0, -10)
  dimension "d103" = 10
  dimension "d104" = 1
  dimension "d105" = 3.2
  dimension "d107" = 360
  constraint coincident L114.end origin
  constraint vertical L114
  constraint tangent L115 A120
  constraint tangent A120 L116
  constraint parallel L115 L116
  constraint tangent L116 A121
  constraint tangent L115 A121
  constraint coincident L114 A120.centre
  constraint parallel L114 L117
  constraint coincident P0 L108.end
  constraint midpoint L117 P0
  measures "d103" distance of L108.start L114.end
  measures "d104" distance of A120.centre P0
  measures "d105" diameter of A120
extrude "Extrude7" cut sketch "Sketch7" against normal blind 5 contours L108 L113 L126 L127 A131 | L108 L113 A130 L126 L127 | L108 L109 L110 L111 L112 L113 L115 A120 L116 L118 L119 A123 L120 L121 A125 L122 L123 A127 L124 L125 A129 L126 L127 A131 | L108 L109 L115 A120 L116 | L108 L109 L115 L116 A121 | L112 L113 A128 L124 L125 | L112 L113 L124 L125 A129 | L109 L110 L118 L119 A123 | L109 L110 A122 L118 L119 | L111 L112 A126 L122 L123 | L111 L112 L122 L123 A127 | L110 L111 L120 L121 A125 | L110 L111 A124 L120 L121 bodies 2
fillet "Fillet10" radius 2.5 12 edges at (-7.0603, 5.9238, 2.5) (-1.6, 9.0762, 2.5) (1.6, 9.0762, 2.5) (7.0603, 5.9238, 2.5) (8.6603, 3.1525, 2.5) (8.6603, -3.1525, 2.5) (7.0603, -5.9238, 2.5) (1.6, -9.0762, 2.5) (-1.6, -9.0762, 2.5) (-7.0603, -5.9238, 2.5) (-8.6603, -3.1525, 2.5) (-8.6603, 3.1525, 2.5) on bodies 2
sketch "Sketch8" plane through (0, 0, 5) normal (0, 0, 1) x (-1, 0, 0)
  arc A0 (8.6603, -1.7091) -> (9.9103, -3.8742) centre (11.1603, -1.7091) ccw
  line L0 (9.9103, -3.8742) -> (10.3263, -4.1144)
  arc A1 (8.7263, -6.8856) -> (10.3263, -4.1144) centre (9.5263, -5.5) ccw
  line L1 (8.7263, -6.8856) -> (8.3103, -6.6454)
  arc A2 (8.3103, -6.6454) -> (5.8103, -6.6454) centre (7.0603, -8.8105) ccw
  line L2 (5.8103, -6.6454) -> (2.85, -8.3546)
  arc A3 (2.85, -8.3546) -> (1.6, -10.5196) centre (4.1, -10.5196) ccw
  line L3 (1.6, -10.5196) -> (1.6, -11)
  arc A4 (-1.6, -11) -> (1.6, -11) centre (0, -11) ccw
  line L4 (-1.6, -11) -> (-1.6, -10.5196)
  arc A5 (-1.6, -10.5196) -> (-2.85, -8.3546) centre (-4.1, -10.5196) ccw
  line L5 (-2.85, -8.3546) -> (-5.8103, -6.6454)
  arc A6 (-5.8103, -6.6454) -> (-8.3103, -6.6454) centre (-7.0603, -8.8105) ccw
  line L6 (-8.3103, -6.6454) -> (-8.7263, -6.8856)
  arc A7 (-10.3263, -4.1144) -> (-8.7263, -6.8856) centre (-9.5263, -5.5) ccw
  line L7 (-10.3263, -4.1144) -> (-9.9103, -3.8742)
  arc A8 (-9.9103, -3.8742) -> (-8.6603, -1.7091) centre (-11.1603, -1.7091) ccw
  line L8 (-8.6603, -1.7091) -> (-8.6603, 1.7091)
  arc A9 (-8.6603, 1.7091) -> (-9.9103, 3.8742) centre (-11.1603, 1.7091) ccw
  line L9 (-9.9103, 3.8742) -> (-10.3263, 4.1144)
  arc A10 (-8.7263, 6.8856) -> (-10.3263, 4.1144) centre (-9.5263, 5.5) ccw
  line L10 (-8.7263, 6.8856) -> (-8.3103, 6.6454)
  arc A11 (-8.3103, 6.6454) -> (-5.8103, 6.6454) centre (-7.0603, 8.8105) ccw
  line L11 (-5.8103, 6.6454) -> (-2.85, 8.3546)
  arc A12 (-2.85, 8.3546) -> (-1.6, 10.5196) centre (-4.1, 10.5196) ccw
  line L12 (-1.6, 10.5196) -> (-1.6, 11)
  arc A13 (1.6, 11) -> (-1.6, 11) centre (0, 11) ccw
  line L13 (1.6, 11) -> (1.6, 10.5196)
  arc A14 (1.6, 10.5196) -> (2.85, 8.3546) centre (4.1, 10.5196) ccw
  line L14 (2.85, 8.3546) -> (5.8103, 6.6454)
  arc A15 (5.8103, 6.6454) -> (8.3103, 6.6454) centre (7.0603, 8.8105) ccw
  line L15 (8.3103, 6.6454) -> (8.7263, 6.8856)
  arc A16 (10.3263, 4.1144) -> (8.7263, 6.8856) centre (9.5263, 5.5) ccw
  line L16 (10.3263, 4.1144) -> (9.9103, 3.8742)
  arc A17 (9.9103, 3.8742) -> (8.6603, 1.7091) centre (11.1603, 1.7091) ccw
  line L17 (8.6603, 1.7091) -> (8.6603, -1.7091)
  line L18 (1, -45.9087) -> (4, -51.1048)
  line L19 (4, -51.1048) -> (3, -52.8369)
  line L20 (3, -52.8369) -> (-3, -52.8369)
  line L21 (-3, -52.8369) -> (-4, -51.1048)
  line L22 (-4, -51.1048) -> (-1, -45.9087)
  line L23 (-1, -45.9087) -> (1, -45.9087)
  arc A18 (-101.6, 90) -> (-98.4, 90) centre (-100, 90) ccw
  line L24 (-101.6, 90) -> (-101.6, 94)
  arc A19 (-98.4, 94) -> (-101.6, 94) centre (-100, 94) ccw
  line L25 (-98.4, 94) -> (-98.4, 90)
  arc A20 (-110, 101.6) -> (-110, 98.4) centre (-110, 100) ccw
  line L26 (-110, 101.6) -> (-106, 101.6)
  arc A21 (-106, 98.4) -> (-106, 101.6) centre (-106, 100) ccw
  line L27 (-106, 98.4) -> (-110, 98.4)
  arc A22 (-90, 98.4) -> (-90, 101.6) centre (-90, 100) ccw
  line L28 (-90, 98.4) -> (-94, 98.4)
  arc A23 (-94, 101.6) -> (-94, 98.4) centre (-94, 100) ccw
  line L29 (-94, 101.6) -> (-90, 101.6)
  circle A24 centre (-100, 100) radius 3
  arc A25 (-98.4, 110) -> (-101.6, 110) centre (-100, 110) ccw
  line L30 (-98.4, 110) -> (-98.4, 106)
  arc A26 (-101.6, 106) -> (-98.4, 106) centre (-100, 106) ccw
  line L31 (-101.6, 106) -> (-101.6, 110)
  arc A27 (-30, -25) -> (-24, -25) centre (-27, -25) ccw
  line L32 (-30, -25) -> (-30, 25)
  arc A28 (-24, 25) -> (-30, 25) centre (-27, 25) ccw
  line L33 (-24, 25) -> (-24, -25)
  arc A29 (-17.7956, -15.5328) -> (-15.5328, -17.7956) centre (-16.6642, -16.6642) ccw
  line L34 (-17.7956, -15.5328) -> (-14.9672, -12.7044)
  arc A30 (-12.7044, -14.9672) -> (-14.9672, -12.7044) centre (-13.8358, -13.8358) ccw
  line L35 (-12.7044, -14.9672) -> (-15.5328, -17.7956)
  line L36 (12.7044, 14.9672) -> (15.5328, 17.7956)
  arc A31 (17.7956, 15.5328) -> (15.5328, 17.7956) centre (16.6642, 16.6642) ccw
  line L37 (17.7956, 15.5328) -> (14.9672, 12.7044)
  arc A32 (12.7044, 14.9672) -> (14.9672, 12.7044) centre (13.8358, 13.8358) ccw
  line L38 (14.9672, -12.7044) -> (17.7956, -15.5328)
  arc A33 (15.5328, -17.7956) -> (17.7956, -15.5328) centre (16.6642, -16.6642) ccw
  line L39 (15.5328, -17.7956) -> (12.7044, -14.9672)
  arc A34 (14.9672, -12.7044) -> (12.7044, -14.9672) centre (13.8358, -13.8358) ccw
  arc A35 (24, -25) -> (30, -25) centre (27, -25) ccw
  line L40 (24, -25) -> (24, 25)
  arc A36 (30, 25) -> (24, 25) centre (27, 25) ccw
  line L41 (30, 25) -> (30, -25)
  line L42 (-14.9672, 12.7044) -> (-17.7956, 15.5328)
  arc A37 (-15.5328, 17.7956) -> (-17.7956, 15.5328) centre (-16.6642, 16.6642) ccw
  line L43 (-15.5328, 17.7956) -> (-12.7044, 14.9672)
  arc A38 (-14.9672, 12.7044) -> (-12.7044, 14.9672) centre (-13.8358, 13.8358) ccw
  line L44 (112.7195, 117.7075) -> (119.1639, 120.4095)
  arc A39 (122.285, 116.8358) -> (119.1639, 120.4095) centre (120.1306, 118.104) ccw
  line L45 (122.285, 116.8358) -> (118.9823, 111.2253)
  arc A40 (116.8279, 109.9935) -> (118.9823, 111.2253) centre (116.8279, 112.4935) ccw
  line L46 (116.8279, 109.9935) -> (113.6861, 109.9935)
  arc A41 (111.1861, 112.4935) -> (113.6861, 109.9935) centre (113.6861, 112.4935) ccw
  line L47 (111.1861, 112.4935) -> (111.1861, 115.4019)
  arc A42 (112.7195, 117.7075) -> (111.1861, 115.4019) centre (113.6861, 115.4019) ccw
  arc A43 (101.6, 110) -> (98.4, 110) centre (100, 110) ccw
  line L48 (101.6, 110) -> (101.6, 106)
  arc A44 (98.4, 106) -> (101.6, 106) centre (100, 106) ccw
  line L49 (98.4, 106) -> (98.4, 110)
  circle A45 centre (100, 100) radius 3
  arc A46 (90, 101.6) -> (90, 98.4) centre (90, 100) ccw
  line L50 (90, 101.6) -> (94, 101.6)
  arc A47 (94, 98.4) -> (94, 101.6) centre (94, 100) ccw
  line L51 (94, 98.4) -> (90, 98.4)
  arc A48 (110, 98.4) -> (110, 101.6) centre (110, 100) ccw
  line L52 (110, 98.4) -> (106, 98.4)
  arc A49 (106, 101.6) -> (106, 98.4) centre (106, 100) ccw
  line L53 (106, 101.6) -> (110, 101.6)
  arc A50 (98.4, 90) -> (101.6, 90) centre (100, 90) ccw
  line L54 (98.4, 90) -> (98.4, 94)
  arc A51 (101.6, 94) -> (98.4, 94) centre (100, 94) ccw
  line L55 (101.6, 94) -> (101.6, 90)
  arc A52 (101.6, -90) -> (98.4, -90) centre (100, -90) ccw
  line L56 (101.6, -90) -> (101.6, -94)
  arc A53 (98.4, -94) -> (101.6, -94) centre (100, -94) ccw
  line L57 (98.4, -94) -> (98.4, -90)
  arc A54 (110, -101.6) -> (110, -98.4) centre (110, -100) ccw
  line L58 (110, -101.6) -> (106, -101.6)
  arc A55 (106, -98.4) -> (106, -101.6) centre (106, -100) ccw
  line L59 (106, -98.4) -> (110, -98.4)
  arc A56 (90, -98.4) -> (90, -101.6) centre (90, -100) ccw
  line L60 (90, -98.4) -> (94, -98.4)
  arc A57 (94, -101.6) -> (94, -98.4) centre (94, -100) ccw
  line L61 (94, -101.6) -> (90, -101.6)
  circle A58 centre (100, -100) radius 3
  arc A59 (98.4, -110) -> (101.6, -110) centre (100, -110) ccw
  line L62 (98.4, -110) -> (98.4, -106)
  arc A60 (101.6, -106) -> (98.4, -106) centre (100, -106) ccw
  line L63 (101.6, -106) -> (101.6, -110)
  line L64 (118.9823, -111.2253) -> (122.285, -116.8358)
  arc A61 (119.1639, -120.4095) -> (122.285, -116.8358) centre (120.1306, -118.104) ccw
  line L65 (119.1639, -120.4095) -> (112.7195, -117.7075)
  arc A62 (111.1861, -115.4019) -> (112.7195, -117.7075) centre (113.6861, -115.4019) ccw
  line L66 (111.1861, -115.4019) -> (111.1861, -112.4935)
  arc A63 (113.6861, -109.9935) -> (111.1861, -112.4935) centre (113.6861, -112.4935) ccw
  line L67 (113.6861, -109.9935) -> (116.8279, -109.9935)
  arc A64 (118.9823, -111.2253) -> (116.8279, -109.9935) centre (116.8279, -112.4935) ccw
  arc A65 (-101.6, -110) -> (-98.4, -110) centre (-100, -110) ccw
  line L68 (-101.6, -110) -> (-101.6, -106)
  arc A66 (-98.4, -106) -> (-101.6, -106) centre (-100, -106) ccw
  line L69 (-98.4, -106) -> (-98.4, -110)
  circle A67 centre (-100, -100) radius 3
  arc A68 (-90, -101.6) -> (-90, -98.4) centre (-90, -100) ccw
  line L70 (-90, -101.6) -> (-94, -101.6)
  arc A69 (-94, -98.4) -> (-94, -101.6) centre (-94, -100) ccw
  line L71 (-94, -98.4) -> (-90, -98.4)
  arc A70 (-110, -98.4) -> (-110, -101.6) centre (-110, -100) ccw
  line L72 (-110, -98.4) -> (-106, -98.4)
  arc A71 (-106, -101.6) -> (-106, -98.4) centre (-106, -100) ccw
  line L73 (-106, -101.6) -> (-110, -101.6)
  arc A72 (-98.4, -90) -> (-101.6, -90) centre (-100, -90) ccw
  line L74 (-98.4, -90) -> (-98.4, -94)
  arc A73 (-101.6, -94) -> (-98.4, -94) centre (-100, -94) ccw
  line L75 (-101.6, -94) -> (-101.6, -90)
  line L76 (-116.8279, -109.9935) -> (-113.6861, -109.9935)
  arc A74 (-111.1861, -112.4935) -> (-113.6861, -109.9935) centre (-113.6861, -112.4935) ccw
  line L77 (-111.1861, -112.4935) -> (-111.1861, -115.4019)
  arc A75 (-112.7195, -117.7075) -> (-111.1861, -115.4019) centre (-113.6861, -115.4019) ccw
  line L78 (-112.7195, -117.7075) -> (-119.1639, -120.4095)
  arc A76 (-122.285, -116.8358) -> (-119.1639, -120.4095) centre (-120.1306, -118.104) ccw
  line L79 (-122.285, -116.8358) -> (-118.9823, -111.2253)
  arc A77 (-116.8279, -109.9935) -> (-118.9823, -111.2253) centre (-116.8279, -112.4935) ccw
  line L80 (-118.9823, 111.2253) -> (-122.285, 116.8358)
  arc A78 (-119.1639, 120.4095) -> (-122.285, 116.8358) centre (-120.1306, 118.104) ccw
  line L81 (-119.1639, 120.4095) -> (-112.7195, 117.7075)
  arc A79 (-111.1861, 115.4019) -> (-112.7195, 117.7075) centre (-113.6861, 115.4019) ccw
  line L82 (-111.1861, 115.4019) -> (-111.1861, 112.4935)
  arc A80 (-113.6861, 109.9935) -> (-111.1861, 112.4935) centre (-113.6861, 112.4935) ccw
  line L83 (-113.6861, 109.9935) -> (-116.8279, 109.9935)
  arc A81 (-118.9823, 111.2253) -> (-116.8279, 109.9935) centre (-116.8279, 112.4935) ccw
  arc A82 (16.6527, -80.0321) -> (19.3611, -77.7595) centre (16.8706, -77.5416) ccw
  line L84 (19.3611, -77.7595) -> (21.3355, -55.1918)
  arc A83 (29.6477, -51.8989) -> (21.3355, -55.1918) centre (26.3165, -55.6276) ccw
  line L85 (29.6477, -51.8989) -> (81.7303, -98.4286)
  arc A84 (86.4985, -105.2878) -> (81.7303, -98.4286) centre (69.7381, -111.852) ccw
  arc A85 (86.4985, -105.2878) -> (94.5518, -113.4375) centre (100, -100) ccw
  line L86 (94.5518, -113.4375) -> (119.1307, -123.403)
  arc A86 (119.1307, -123.403) -> (125.4028, -116.3824) centre (121.0094, -118.7694) ccw
  line L87 (125.4028, -116.3824) -> (112.7409, -93.0776)
  arc A87 (112.7409, -93.0776) -> (103.7386, -85.9903) centre (100, -100) ccw
  arc A88 (96.3875, -82.0222) -> (103.7386, -85.9903) centre (108.3797, -68.5989) ccw
  line L88 (96.3875, -82.0222) -> (44.6753, -35.8235)
  arc A89 (38, -20.9087) -> (44.6753, -35.8235) centre (58, -20.9087) ccw
  line L89 (38, -20.9087) -> (38, 20.9087)
  arc A90 (44.6753, 35.8235) -> (38, 20.9087) centre (58, 20.9087) ccw
  line L90 (44.6753, 35.8235) -> (96.3875, 82.0222)
  arc A91 (103.7386, 85.9903) -> (96.3875, 82.0222) centre (108.3797, 68.5989) ccw
  arc A92 (103.7386, 85.9903) -> (112.7409, 93.0776) centre (100, 100) ccw
  line L91 (112.7409, 93.0776) -> (125.4028, 116.3824)
  arc A93 (125.4028, 116.3824) -> (119.1307, 123.403) centre (121.0094, 118.7694) ccw
  line L92 (119.1307, 123.403) -> (94.5518, 113.4375)
  arc A94 (94.5518, 113.4375) -> (86.4985, 105.2878) centre (100, 100) ccw
  arc A95 (81.7303, 98.4286) -> (86.4985, 105.2878) centre (69.7381, 111.852) ccw
  line L93 (81.7303, 98.4286) -> (29.156, 51.4596)
  arc A96 (20.8759, 54.4751) -> (29.156, 51.4596) centre (25.8248, 55.1883) ccw
  line L94 (20.8759, 54.4751) -> (16.1217, 87.466)
  arc A97 (16.1217, 87.466) -> (14.4465, 90.5321) centre (11.1729, 86.7528) ccw
  line L95 (14.4465, 90.5321) -> (10.4093, 94.0293)
  arc A98 (10.4093, 94.0293) -> (7.1356, 95.25) centre (7.1356, 90.25) ccw
  line L96 (7.1356, 95.25) -> (-7.1356, 95.25)
  arc A99 (-7.1356, 95.25) -> (-10.4093, 94.0293) centre (-7.1356, 90.25) ccw
  line L97 (-10.4093, 94.0293) -> (-14.4465, 90.5321)
  arc A100 (-14.4465, 90.5321) -> (-16.1217, 87.466) centre (-11.1729, 86.7528) ccw
  line L98 (-16.1217, 87.466) -> (-20.8759, 54.4751)
  arc A101 (-29.156, 51.4596) -> (-20.8759, 54.4751) centre (-25.8248, 55.1883) ccw
  line L99 (-29.156, 51.4596) -> (-81.7303, 98.4286)
  arc A102 (-86.4985, 105.2878) -> (-81.7303, 98.4286) centre (-69.7381, 111.852) ccw
  arc A103 (-86.4985, 105.2878) -> (-94.5518, 113.4375) centre (-100, 100) ccw
  line L100 (-94.5518, 113.4375) -> (-119.1307, 123.403)
  arc A104 (-119.1307, 123.403) -> (-125.4028, 116.3824) centre (-121.0094, 118.7694) ccw
  line L101 (-125.4028, 116.3824) -> (-112.7409, 93.0776)
  arc A105 (-112.7409, 93.0776) -> (-103.7386, 85.9903) centre (-100, 100) ccw
  arc A106 (-96.3875, 82.0222) -> (-103.7386, 85.9903) centre (-108.3797, 68.5989) ccw
  line L102 (-96.3875, 82.0222) -> (-44.6753, 35.8235)
  arc A107 (-38, 20.9087) -> (-44.6753, 35.8235) centre (-58, 20.9087) ccw
  line L103 (-38, 20.9087) -> (-38, -20.9087)
  arc A108 (-44.6753, -35.8235) -> (-38, -20.9087) centre (-58, -20.9087) ccw
  line L104 (-44.6753, -35.8235) -> (-96.3875, -82.0222)
  arc A109 (-103.7386, -85.9903) -> (-96.3875, -82.0222) centre (-108.3797, -68.5989) ccw
  arc A110 (-103.7386, -85.9903) -> (-112.7409, -93.0776) centre (-100, -100) ccw
  line L105 (-112.7409, -93.0776) -> (-125.4028, -116.3824)
  arc A111 (-125.4028, -116.3824) -> (-119.1307, -123.403) centre (-121.0094, -118.7694) ccw
  line L106 (-119.1307, -123.403) -> (-94.5518, -113.4375)
  arc A112 (-94.5518, -113.4375) -> (-86.4985, -105.2878) centre (-100, -100) ccw
  arc A113 (-81.7303, -98.4286) -> (-86.4985, -105.2878) centre (-69.7381, -111.852) ccw
  line L107 (-81.7303, -98.4286) -> (-29.6477, -51.8989)
  arc A114 (-21.3355, -55.1918) -> (-29.6477, -51.8989) centre (-26.3165, -55.6276) ccw
  line L108 (-21.3355, -55.1918) -> (-19.3611, -77.7595)
  arc A115 (-19.3611, -77.7595) -> (-16.6527, -80.0321) centre (-16.8706, -77.5416) ccw
  line L109 (-16.6527, -80.0321) -> (-12.2821, -79.6497)
  arc A116 (-12.2821, -79.6497) -> (-10.0175, -77.4546) centre (-12.5, -77.1592) ccw
  arc A117 (-7.535, -75.25) -> (-10.0175, -77.4546) centre (-7.535, -77.75) ccw
  line L110 (-7.535, -75.25) -> (7.535, -75.25)
  arc A118 (10.0175, -77.4546) -> (7.535, -75.25) centre (7.535, -77.75) ccw
  arc A119 (10.0175, -77.4546) -> (12.2821, -79.6497) centre (12.5, -77.1592) ccw
  line L111 (12.2821, -79.6497) -> (16.6527, -80.0321)
  line L112 (26, 35.4) -> (18, 35.4)
  arc A120 (18, 38.6) -> (18, 35.4) centre (18, 37) ccw
  line L113 (18, 38.6) -> (26, 38.6)
  arc A121 (26, 35.4) -> (26, 38.6) centre (26, 37) ccw
  circle A122 centre (14.8248, -75.7565) radius 1.6
  line L114 (-5, -61.3002) -> (5, -61.3002)
  arc A123 (5, -71.3002) -> (5, -61.3002) centre (5, -66.3002) ccw
  line L115 (5, -71.3002) -> (-5, -71.3002)
  arc A124 (-5, -61.3002) -> (-5, -71.3002) centre (-5, -66.3002) ccw
  circle A125 centre (16.4789, -56.85) radius 1.6
  line L116 (10, 39) -> (10, 36)
  arc A126 (4, 30) -> (10, 36) centre (4, 36) ccw
  line L117 (4, 30) -> (-4, 30)
  arc A127 (-10, 36) -> (-4, 30) centre (-4, 36) ccw
  line L118 (-10, 36) -> (-10, 39)
  arc A128 (-4, 45) -> (-10, 39) centre (-4, 39) ccw
  line L119 (-4, 45) -> (4, 45)
  arc A129 (10, 39) -> (4, 45) centre (4, 39) ccw
  line L120 (-26, 38.6) -> (-18, 38.6)
  arc A130 (-18, 35.4) -> (-18, 38.6) centre (-18, 37) ccw
  line L121 (-18, 35.4) -> (-26, 35.4)
  arc A131 (-26, 38.6) -> (-26, 35.4) centre (-26, 37) ccw
  circle A132 centre (-14.8248, -75.7565) radius 1.6
  line L122 (-12.5, -35.4) -> (12.5, -35.4)
  arc A133 (12.5, -38.6) -> (12.5, -35.4) centre (12.5, -37) ccw
  line L123 (12.5, -38.6) -> (-12.5, -38.6)
  arc A134 (-12.5, -35.4) -> (-12.5, -38.6) centre (-12.5, -37) ccw
  circle A135 centre (-16.4789, -56.85) radius 1.6
  line L124 (6, 80.25) -> (6, 60.25)
  arc A136 (-6, 60.25) -> (6, 60.25) centre (0, 60.25) ccw
  line L125 (-6, 60.25) -> (-6, 80.25)
  arc A137 (6, 80.25) -> (-6, 80.25) centre (0, 80.25) ccw
  line L126 (12.4279, 92.2807) -> (4.9473, 83.6448) construction
  line L127 (-12.4279, 92.2807) -> (-4.9473, 83.6448) construction
  circle A138 centre (8.6876, 87.9627) radius 1.6
  circle A139 centre (-8.6876, 87.9627) radius 1.6
  line L128 (20.8759, 54.4751) -> (6, 60.25) construction
  line L129 (-6, 60.25) -> (-20.8759, 54.4751) construction
  line L130 (16.0316, 37) -> (8.6876, 87.9627) construction
  line L131 (18, 37) -> (10, 37) construction
  line L132 (15.5165, 51.7922) -> (13.8049, 63.6695)
  arc A140 (13.8049, 63.6695) -> (10.6376, 63.2131) centre (12.2213, 63.4413) ccw
  line L133 (10.6376, 63.2131) -> (12.3492, 51.3358)
  arc A141 (12.3492, 51.3358) -> (15.5165, 51.7922) centre (13.9329, 51.564) ccw
  line L134 (13.9329, 51.564) -> (12.2213, 63.4413) construction
  line L135 (0, 60.25) -> (0, 80.25) construction
  arc A142 (-15.5165, 51.7922) -> (-12.3492, 51.3358) centre (-13.9329, 51.564) ccw
  line L136 (-10.6376, 63.2131) -> (-12.3492, 51.3358)
  line L137 (-15.5165, 51.7922) -> (-13.8049, 63.6695)
  arc A143 (-10.6376, 63.2131) -> (-13.8049, 63.6695) centre (-12.2213, 63.4413) ccw
  point P0 (13.0771, 57.5027)
  dimension "d112" = 3.2
  dimension "d113" = 3.2
  dimension "d114" = 6
  dimension "d115" = 3.2
  constraint midpoint L95 L126.start
  constraint coincident A137 L126.end
  constraint perpendicular L95 L126
  constraint midpoint L97 L127.start
  constraint coincident A137 L127.end
  constraint perpendicular L97 L127
  constraint midpoint L126 A138.centre
  constraint midpoint L127 A139.centre
  constraint coincident A96.start L94.start
  constraint coincident L124.end A136.end
  constraint coincident A136.start L125.start
  constraint coincident L98.end A101.end
  constraint coincident A138.centre L130.end
  constraint parallel L94 L130
  constraint coincident A120.centre L131.start
  constraint coincident L116 L131.end
  constraint perpendicular L116 L131
  constraint coincident L130.start L131
  constraint tangent L132 A140
  constraint tangent A140 L133
  constraint parallel L132 L133
  constraint tangent L133 A141
  constraint tangent L132 A141
  constraint coincident L130 A140.centre
  constraint parallel L130 L134
  constraint coincident L130 P0
  constraint coincident L128 P0
  constraint midpoint L134 P0
  constraint coincident A136.centre L135.start
  constraint coincident A137.centre L135.end
  constraint symmetric L132.start L135 A142.start
  constraint symmetric L132.end L135 L137.end
  constraint symmetric A140.end L135 L136.start